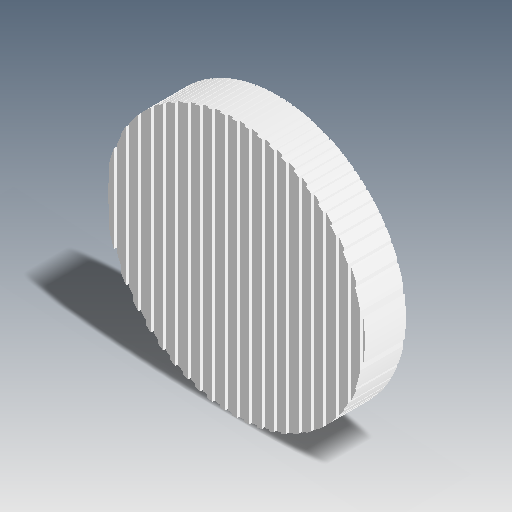
# Autodesk Inventor part: Polarizer
Saved by Autodesk Inventor 2026 (Build 300175050, 175E)
## iProperties
Created: 2025-08-02
Part Number: Polarizer
Material: Generic
Document SubType Name: Modeling
Designer: aman0
Density: 1 g/cm^3
Appearance: Default
Author: aman0
Autodesk Inventor part; units mm, degrees
ref_plane "YZ Plane" through (0, 0, 0) normal (1, 0, 0) x (0, 1, 0)
ref_plane "XZ Plane" through (0, 0, 0) normal (0, 1, 0) x (-1, 0, 0)
ref_plane "XY Plane" through (0, 0, 0) normal (0, 0, 1) x (1, 0, 0)
sketch "Sketch1" plane through (0, 0, 0) normal (0, 0, 1) x (1, 0, 0)
  circle A0 centre (0, 0) radius 12.5
  line L0 (-0.25, -12.5) -> (0.25, -12.5)
  line L1 (0.25, -12.5) -> (0.25, 12.5)
  line L2 (0.25, 12.5) -> (-0.25, 12.5)
  line L3 (-0.25, 12.5) -> (-0.25, -12.5)
  line L4 (-0.25, -12.5) -> (0.25, 12.5) construction
  line L5 (0.25, -12.5) -> (-0.25, 12.5) construction
  line L6 (-0.85, 12.5) -> (-0.85, -12.5)
  line L7 (-0.35, -12.5) -> (-0.35, 12.5)
  line L8 (0.35, 12.5) -> (0.35, -12.5)
  line L9 (0.85, -12.5) -> (0.85, 12.5)
  line L10 (-1.45, 12.5) -> (-1.45, -12.5)
  line L11 (-0.95, -12.5) -> (-0.95, 12.5)
  line L12 (0.95, 12.5) -> (0.95, -12.5)
  line L13 (1.45, -12.5) -> (1.45, 12.5)
  line L14 (-2.05, 12.5) -> (-2.05, -12.5)
  line L15 (-1.55, -12.5) -> (-1.55, 12.5)
  line L16 (1.55, 12.5) -> (1.55, -12.5)
  line L17 (2.05, -12.5) -> (2.05, 12.5)
  line L18 (-2.65, 12.5) -> (-2.65, -12.5)
  line L19 (-2.15, -12.5) -> (-2.15, 12.5)
  line L20 (2.15, 12.5) -> (2.15, -12.5)
  line L21 (2.65, -12.5) -> (2.65, 12.5)
  line L22 (-3.25, 12.5) -> (-3.25, -12.5)
  line L23 (-2.75, -12.5) -> (-2.75, 12.5)
  line L24 (2.75, 12.5) -> (2.75, -12.5)
  line L25 (3.25, -12.5) -> (3.25, 12.5)
  line L26 (-3.85, 12.5) -> (-3.85, -12.5)
  line L27 (-3.35, -12.5) -> (-3.35, 12.5)
  line L28 (3.35, 12.5) -> (3.35, -12.5)
  line L29 (3.85, -12.5) -> (3.85, 12.5)
  line L30 (-4.45, 12.5) -> (-4.45, -12.5)
  line L31 (-3.95, -12.5) -> (-3.95, 12.5)
  line L32 (3.95, 12.5) -> (3.95, -12.5)
  line L33 (4.45, -12.5) -> (4.45, 12.5)
  line L34 (-5.05, 12.5) -> (-5.05, -12.5)
  line L35 (-4.55, -12.5) -> (-4.55, 12.5)
  line L36 (4.55, 12.5) -> (4.55, -12.5)
  line L37 (5.05, -12.5) -> (5.05, 12.5)
  line L38 (-5.65, 12.5) -> (-5.65, -12.5)
  line L39 (-5.15, -12.5) -> (-5.15, 12.5)
  line L40 (5.15, 12.5) -> (5.15, -12.5)
  line L41 (5.65, -12.5) -> (5.65, 12.5)
  line L42 (-6.25, 12.5) -> (-6.25, -12.5)
  line L43 (-5.75, -12.5) -> (-5.75, 12.5)
  line L44 (5.75, 12.5) -> (5.75, -12.5)
  line L45 (6.25, -12.5) -> (6.25, 12.5)
  line L46 (-6.85, 12.5) -> (-6.85, -12.5)
  line L47 (-6.35, -12.5) -> (-6.35, 12.5)
  line L48 (6.35, 12.5) -> (6.35, -12.5)
  line L49 (6.85, -12.5) -> (6.85, 12.5)
  line L50 (-7.45, 12.5) -> (-7.45, -12.5)
  line L51 (-6.95, -12.5) -> (-6.95, 12.5)
  line L52 (6.95, 12.5) -> (6.95, -12.5)
  line L53 (7.45, -12.5) -> (7.45, 12.5)
  line L54 (-8.05, 12.5) -> (-8.05, -12.5)
  line L55 (-7.55, -12.5) -> (-7.55, 12.5)
  line L56 (7.55, 12.5) -> (7.55, -12.5)
  line L57 (8.05, -12.5) -> (8.05, 12.5)
  line L58 (-8.65, 12.5) -> (-8.65, -12.5)
  line L59 (-8.15, -12.5) -> (-8.15, 12.5)
  line L60 (8.15, 12.5) -> (8.15, -12.5)
  line L61 (8.65, -12.5) -> (8.65, 12.5)
  line L62 (-9.25, 12.5) -> (-9.25, -12.5)
  line L63 (-8.75, -12.5) -> (-8.75, 12.5)
  line L64 (8.75, 12.5) -> (8.75, -12.5)
  line L65 (9.25, -12.5) -> (9.25, 12.5)
  line L66 (-9.85, 12.5) -> (-9.85, -12.5)
  line L67 (-9.35, -12.5) -> (-9.35, 12.5)
  line L68 (9.35, 12.5) -> (9.35, -12.5)
  line L69 (9.85, -12.5) -> (9.85, 12.5)
  line L70 (-10.45, 12.5) -> (-10.45, -12.5)
  line L71 (-9.95, -12.5) -> (-9.95, 12.5)
  line L72 (9.95, 12.5) -> (9.95, -12.5)
  line L73 (10.45, -12.5) -> (10.45, 12.5)
  line L74 (-11.05, 12.5) -> (-11.05, -12.5)
  line L75 (-10.55, -12.5) -> (-10.55, 12.5)
  line L76 (10.55, 12.5) -> (10.55, -12.5)
  line L77 (11.05, -12.5) -> (11.05, 12.5)
  line L78 (-11.65, 12.5) -> (-11.65, -12.5)
  line L79 (-11.15, -12.5) -> (-11.15, 12.5)
  line L80 (11.15, 12.5) -> (11.15, -12.5)
  line L81 (11.65, -12.5) -> (11.65, 12.5)
  line L82 (-12.25, 12.5) -> (-12.25, -12.5)
  line L83 (-11.75, -12.5) -> (-11.75, 12.5)
  line L84 (11.75, 12.5) -> (11.75, -12.5)
  line L85 (12.25, -12.5) -> (12.25, 12.5)
  line L86 (-12.85, 12.5) -> (-12.85, -12.5)
  line L87 (-12.35, -12.5) -> (-12.35, 12.5)
  line L88 (12.35, 12.5) -> (12.35, -12.5)
  line L89 (12.85, -12.5) -> (12.85, 12.5)
  line L90 (-13.45, 12.5) -> (-13.45, -12.5)
  line L91 (-12.95, -12.5) -> (-12.95, 12.5)
  line L92 (12.95, 12.5) -> (12.95, -12.5)
  line L93 (13.45, -12.5) -> (13.45, 12.5)
  line L94 (-14.05, 12.5) -> (-14.05, -12.5)
  line L95 (-13.55, -12.5) -> (-13.55, 12.5)
  line L96 (13.55, 12.5) -> (13.55, -12.5)
  line L97 (14.05, -12.5) -> (14.05, 12.5)
  line L98 (-14.65, 12.5) -> (-14.65, -12.5)
  line L99 (-14.15, -12.5) -> (-14.15, 12.5)
  line L100 (14.15, 12.5) -> (14.15, -12.5)
  line L101 (14.65, -12.5) -> (14.65, 12.5)
  line L102 (-15.25, 12.5) -> (-15.25, -12.5)
  line L103 (-14.75, -12.5) -> (-14.75, 12.5)
  point P0 (12.35, 1.9307)
  point P1 (12.35, -1.9307)
  point P2 (11.65, -4.5307)
  point P3 (11.65, 4.5307)
  point P4 (11.15, 5.6504)
  point P5 (11.15, -5.6504)
  point P6 (10.45, -6.8591)
  point P7 (10.45, 6.8591)
  point P8 (9.95, 7.5662)
  point P9 (9.95, -7.5662)
  point P10 (9.25, -8.4076)
  point P11 (9.25, 8.4076)
  point P12 (8.75, 8.9268)
  point P13 (8.75, -8.9268)
  point P14 (8.05, -9.5628)
  point P15 (8.05, 9.5628)
  point P16 (7.55, 9.9623)
  point P17 (7.55, -9.9623)
  point P18 (6.85, -10.456)
  point P19 (6.85, 10.456)
  point P20 (6.35, 10.767)
  point P21 (6.35, -10.767)
  point P22 (5.65, -11.1502)
  point P23 (5.65, 11.1502)
  point P24 (5.15, 11.3898)
  point P25 (5.15, -11.3898)
  point P26 (4.45, -11.6811)
  point P27 (4.45, 11.6811)
  point P28 (3.95, 11.8595)
  point P29 (3.95, -11.8595)
  point P30 (3.25, -12.0701)
  point P31 (3.25, 12.0701)
  point P32 (2.75, 12.1937)
  point P33 (2.75, -12.1937)
  point P34 (2.05, -12.3308)
  point P35 (2.05, 12.3308)
  point P36 (1.55, 12.4035)
  point P37 (1.55, -12.4035)
  point P38 (0.85, -12.4711)
  point P39 (0.85, 12.4711)
  point P40 (0.35, 12.4951)
  point P41 (0.35, -12.4951)
  point P42 (-0.35, -12.4951)
  point P43 (-0.35, 12.4951)
  point P44 (-0.85, 12.4711)
  point P45 (-0.85, -12.4711)
  point P46 (-1.55, -12.4035)
  point P47 (-1.55, 12.4035)
  point P48 (-2.05, 12.3308)
  point P49 (-2.05, -12.3308)
  point P50 (-2.75, -12.1937)
  point P51 (-2.75, 12.1937)
  point P52 (-3.25, 12.0701)
  point P53 (-3.25, -12.0701)
  point P54 (-3.95, -11.8595)
  point P55 (-3.95, 11.8595)
  point P56 (-4.45, 11.6811)
  point P57 (-4.45, -11.6811)
  point P58 (-5.15, -11.3898)
  point P59 (-5.15, 11.3898)
  point P60 (-5.65, 11.1502)
  point P61 (-5.65, -11.1502)
  point P62 (-6.35, -10.767)
  point P63 (-6.35, 10.767)
  point P64 (-6.85, 10.456)
  point P65 (-6.85, -10.456)
  point P66 (-7.55, -9.9623)
  point P67 (-7.55, 9.9623)
  point P68 (-8.05, 9.5628)
  point P69 (-8.05, -9.5628)
  point P70 (-8.75, -8.9268)
  point P71 (-8.75, 8.9268)
  point P72 (-9.25, 8.4076)
  point P73 (-9.25, -8.4076)
  point P74 (-9.95, -7.5662)
  point P75 (-9.95, 7.5662)
  point P76 (-10.45, 6.8591)
  point P77 (-10.45, -6.8591)
  point P78 (-11.15, -5.6504)
  point P79 (-11.15, 5.6504)
  point P80 (-11.65, 4.5307)
  point P81 (-11.65, -4.5307)
  point P82 (-12.35, -1.9307)
  point P83 (-12.35, 1.9307)
  point P84 (12.25, -2.4875)
  point P85 (12.25, 2.4875)
  point P86 (11.75, 4.2647)
  point P87 (11.75, -4.2647)
  point P88 (11.05, -5.8436)
  point P89 (11.05, 5.8436)
  point P90 (10.55, 6.7043)
  point P91 (10.55, -6.7043)
  point P92 (9.85, -7.6959)
  point P93 (9.85, 7.6959)
  point P94 (9.35, 8.2962)
  point P95 (9.35, -8.2962)
  point P96 (8.65, -9.0237)
  point P97 (8.65, 9.0237)
  point P98 (8.15, 9.4777)
  point P99 (8.15, -9.4777)
  point P100 (7.45, -10.0373)
  point P101 (7.45, 10.0373)
  point P102 (6.95, 10.3898)
  point P103 (6.95, -10.3898)
  point P104 (6.25, -10.8253)
  point P105 (6.25, 10.8253)
  point P106 (5.75, 11.099)
  point P107 (5.75, -11.099)
  point P108 (5.05, -11.4345)
  point P109 (5.05, 11.4345)
  point P110 (4.55, 11.6425)
  point P111 (4.55, -11.6425)
  point P112 (3.85, -11.8923)
  point P113 (3.85, 11.8923)
  point P114 (3.35, 12.0427)
  point P115 (3.35, -12.0427)
  point P116 (2.65, -12.2159)
  point P117 (2.65, 12.2159)
  point P118 (2.15, 12.3137)
  point P119 (2.15, -12.3137)
  point P120 (1.45, -12.4156)
  point P121 (1.45, 12.4156)
  point P122 (0.95, 12.4638)
  point P123 (0.95, -12.4638)
  point P124 (-0.25, 12.4975)
  point P125 (-0.25, -12.4975)
  point P126 (0.25, -12.4975)
  point P127 (0.25, 12.4975)
  point P128 (-0.95, -12.4638)
  point P129 (-0.95, 12.4638)
  point P130 (-1.45, 12.4156)
  point P131 (-1.45, -12.4156)
  point P132 (-2.15, -12.3137)
  point P133 (-2.15, 12.3137)
  point P134 (-2.65, 12.2159)
  point P135 (-2.65, -12.2159)
  point P136 (-3.35, -12.0427)
  point P137 (-3.35, 12.0427)
  point P138 (-3.85, 11.8923)
  point P139 (-3.85, -11.8923)
  point P140 (-4.55, -11.6425)
  point P141 (-4.55, 11.6425)
  point P142 (-5.05, 11.4345)
  point P143 (-5.05, -11.4345)
  point P144 (-5.75, -11.099)
  point P145 (-5.75, 11.099)
  point P146 (-6.25, 10.8253)
  point P147 (-6.25, -10.8253)
  point P148 (-6.95, -10.3898)
  point P149 (-6.95, 10.3898)
  point P150 (-7.45, 10.0373)
  point P151 (-7.45, -10.0373)
  point P152 (-8.15, -9.4777)
  point P153 (-8.15, 9.4777)
  point P154 (-8.65, 9.0237)
  point P155 (-8.65, -9.0237)
  point P156 (-9.35, -8.2962)
  point P157 (-9.35, 8.2962)
  point P158 (-9.85, 7.6959)
  point P159 (-9.85, -7.6959)
  point P160 (-10.55, -6.7043)
  point P161 (-10.55, 6.7043)
  point P162 (-11.05, 5.8436)
  point P163 (-11.05, -5.8436)
  point P164 (-11.75, -4.2647)
  point P165 (-11.75, 4.2647)
  point P166 (-12.25, 2.4875)
  point P167 (-12.25, -2.4875)
  dimension "d0" = 25
  dimension "d1" = 0.5
  dimension "d2" = 25
  dimension "d5" = 0.6
  constraints: 208 end point, 2 horizontal, 2 midpoint, 2 parallel, 1 coincident, 1 perpendicular, 295 other
  measures "d1" distance of L0.start L0.end
  measures "d2" distance of L1.end L0.end
  measures "d5" distance of L2.end L6.start
extrude "Extrusion1" add sketch "Sketch1" along normal blind 4 contours A0 L88 | L81 A0 L80 | L73 A0 L72 | L65 A0 L64 | L57 A0 L56 | L49 A0 L48 | L41 A0 L40 | L33 A0 L32 | L25 A0 L24 | L17 A0 L16 | L9 A0 L8 | L7 A0 L6 | L15 A0 L14 | L23 A0 L22 | L31 A0 L30 | L39 A0 L38 | L47 A0 L46 | L55 A0 L54 | L63 A0 L62 | L71 A0 L70 | L79 A0 L78 | L87 A0
extrude "Extrusion2" add sketch "Sketch1" along normal blind 4.2 contours L85 A0 L84 | L77 A0 L76 | L69 A0 L68 | L61 A0 L60 | L53 A0 L52 | L45 A0 L44 | L37 A0 L36 | L29 A0 L28 | L21 A0 L20 | L13 A0 L12 | L1 A0 L3 | L11 A0 L10 | L19 A0 L18 | L27 A0 L26 | L35 A0 L34 | L43 A0 L42 | L51 A0 L50 | L59 A0 L58 | L67 A0 L66 | L75 A0 L74 | L83 A0 L82
body "Solid1"
